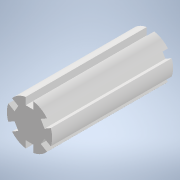
# Autodesk Inventor part: innerShaft
Saved by Autodesk Inventor 2021 (Build 250183000, 183)
## iProperties
Created: 2020-06-26
Part Number: innerShaft
Material: PET Plastic
Document SubType Name: Modeling
Designer: robst
Density: 1.541 g/cm^3
Appearance: Smooth - Yellow
Author: robst
Autodesk Inventor part; units mm, degrees
ref_plane "YZ Plane" through (0, 0, 0) normal (1, 0, 0) x (0, 1, 0)
ref_plane "XZ Plane" through (0, 0, 0) normal (0, 1, 0) x (-1, 0, 0)
ref_plane "XY Plane" through (0, 0, 0) normal (0, 0, 1) x (1, 0, 0)
sketch "Sketch1" plane through (0, 0, 0) normal (0, 0, 1) x (1, 0, 0)
  line L0 (0, 0) -> (0, 9.525) construction
  line L1 (0, 6.35) -> (1.5875, 6.35)
  line L2 (1.5875, 6.35) -> (1.5875, 9.3918)
  line L3 (0, 6.35) -> (-1.5875, 6.35)
  line L4 (-1.5875, 6.35) -> (-1.5875, 9.3918)
  line L5 (-6.293, 1.8002) -> (-8.9273, 3.3211)
  line L6 (-5.4993, 3.175) -> (-6.293, 1.8002)
  line L7 (-5.4993, 3.175) -> (-4.7055, 4.5498)
  line L8 (-4.7055, 4.5498) -> (-7.3398, 6.0707)
  line L9 (-4.7055, -4.5498) -> (-7.3398, -6.0707)
  line L10 (-5.4993, -3.175) -> (-4.7055, -4.5498)
  line L11 (-5.4993, -3.175) -> (-6.293, -1.8002)
  line L12 (-6.293, -1.8002) -> (-8.9273, -3.3211)
  line L13 (1.5875, -6.35) -> (1.5875, -9.3918)
  line L14 (0, -6.35) -> (1.5875, -6.35)
  line L15 (0, -6.35) -> (-1.5875, -6.35)
  line L16 (-1.5875, -6.35) -> (-1.5875, -9.3918)
  line L17 (6.293, -1.8002) -> (8.9273, -3.3211)
  line L18 (5.4993, -3.175) -> (6.293, -1.8002)
  line L19 (5.4993, -3.175) -> (4.7055, -4.5498)
  line L20 (4.7055, -4.5498) -> (7.3398, -6.0707)
  line L21 (4.7055, 4.5498) -> (7.3398, 6.0707)
  line L22 (5.4993, 3.175) -> (4.7055, 4.5498)
  line L23 (5.4993, 3.175) -> (6.293, 1.8002)
  line L24 (6.293, 1.8002) -> (8.9273, 3.3211)
  arc A0 (-1.5875, 9.3918) -> (-7.3398, 6.0707) centre (0, 0) ccw
  arc A1 (-8.9273, 3.3211) -> (-8.9273, -3.3211) centre (0, 0) ccw
  arc A2 (-7.3398, -6.0707) -> (-1.5875, -9.3918) centre (0, 0) ccw
  arc A3 (1.5875, -9.3918) -> (7.3398, -6.0707) centre (0, 0) ccw
  arc A4 (8.9273, -3.3211) -> (8.9273, 3.3211) centre (0, 0) ccw
  arc A5 (7.3398, 6.0707) -> (1.5875, 9.3918) centre (0, 0) ccw
  dimension "splineDepth" = 3.175
  dimension "splineWidth" = 3.175
  dimension "d6" = 360
  constraints: 50 end point, 12 point on circle, 6 centre point, 2 horizontal, 2 perpendicular, 1 coincident, 1 collinear, 1 point on line, 1 vertical, 55 other
  measures "splineDepth" distance from line of L1 L0.end
  measures "splineWidth" distance between parallel lines of L2 L4
extrude "Extrusion1" add sketch "Sketch1" against normal blind 50.8
sketch "Sketch2" plane through (0, 0, -50.8) normal (0, 0, -1) x (-1, 0, 0)
  circle A0 centre (0, 0) radius 6.35
  dimension "innerDiameter" = 12.7
  constraints: 1 centre point, 1 coincident
  measures "innerDiameter" diameter of A0
extrude "Extrusion2" add sketch "Sketch2" along normal blind 50.8
sketch "Sketch3" plane through (0, 0, 0) normal (0, 0, 1) x (1, 0, 0)
  circle A0 centre (0, 0) radius 6.35
  dimension "d13" = 12.7
  constraints: 1 centre point, 1 coincident
  measures "d13" diameter of A0
extrude "Extrusion3" add sketch "Sketch3" along normal blind 50.8
equation "\"d13\" = innerDiameter"
body "Solid1"
